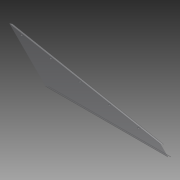
# Autodesk Inventor part: Hopper Back Wedge Side
Saved by Autodesk Inventor 2014 SP1 (Build 180222100, 222)
## iProperties
Created: 2013-12-16
Part Number: Hopper Back Wedge Side
Material: Polycarbonate, Clear
Document SubType Name: Modeling
Designer: Moses
Mass: 66.3982 g
Surface Area: 377.579 cm^2
Volume: 55.3318 cm^3
Density: 1.2 g/cm^3
Appearance: Polycarbonate - Clear
Author: Moses
Autodesk Inventor part; units mm, degrees
ref_plane "YZ Plane" through (0, 0, 0) normal (1, 0, 0) x (0, 1, 0)
ref_plane "XZ Plane" through (0, 0, 0) normal (0, 1, 0) x (-1, 0, 0)
ref_plane "XY Plane" through (0, 0, 0) normal (0, 0, 1) x (1, 0, 0)
sketch "Sketch1" plane through (0, 0, 0) normal (0, 0, 1) x (1, 0, 0)
  line L0 (0, 0) -> (0, 88.9)
  line L1 (0, 88.9) -> (366.2791, 19.3046)
  line L2 (467.8791, 0) -> (366.2791, 0) construction
  line L3 (366.2791, 0) -> (366.2791, 19.3046)
  line L4 (366.2791, 19.3046) -> (467.8791, 0) construction
  line L5 (366.2791, 0) -> (0, 0)
  line L6 (0, 6.35) -> (366.2791, 6.35)
  circle A0 centre (4.3656, 73.025) radius 1.5875 projected
  circle A1 centre (4.3656, 9.525) radius 1.5875 projected
  line L7 (11.9063, 82.55) -> (-3.9687, 82.55) construction
  line L8 (11.9063, 82.55) -> (11.9063, 0) construction
  line L9 (-3.9687, 0) -> (11.9063, 0) construction
  line L10 (-3.9687, 82.55) -> (-3.9687, 0) construction
  circle A2 centre (293.5291, 28.6839) radius 1.5875 projected
  circle A3 centre (161.2752, 53.8129) radius 1.5875 projected
  circle A4 centre (29.0214, 78.942) radius 1.5875 projected
  circle A5 centre (95.1483, 66.3775) radius 1.5875 projected
  circle A6 centre (227.4022, 41.2484) radius 1.5875 projected
  circle A7 centre (359.656, 16.1193) radius 1.5875 projected
  line L11 (21.2196, 88.9079) -> (18.2563, 73.3119) construction
  line L12 (21.2196, 88.9079) -> (370.5693, 22.5292) construction
  line L13 (367.606, 6.9333) -> (370.5693, 22.5292) construction
  line L14 (18.2563, 73.3119) -> (367.606, 6.9333) construction
  dimension "d0" = 88.9
  dimension "d1" = 476.25
  dimension "d5" = 101.6
  dimension "d6" = 6.35
  constraints: 14 end point, 2 perpendicular, 2 point on line, 2 vertical, 1 coincident, 1 collinear, 1 horizontal
  measures "d0" distance of L0.start L0.end
  measures "d1" distance of L0.end L2.start
  measures "d5" distance from line of L2.start L3
  measures "d6" distance between parallel lines of L5 L6
extrude "Extrusion1" add sketch "Sketch1" along normal blind 3.175 contours L0 L1 L3 L6
body "Solid1"
